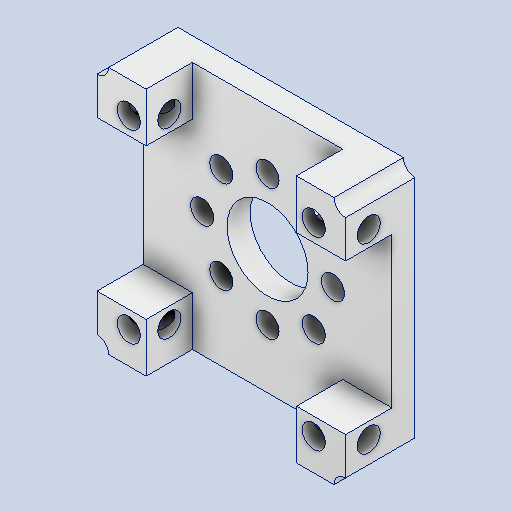
# Autodesk Inventor part: ShoulderMotorMount
Saved by Autodesk Inventor 2023 (Build 270158000, 158)
## iProperties
Created: 2021-01-26
Part Number: ShoulderMotorMount
Material: Aluminum 6061
Document SubType Name: Modeling
Designer: valer
Density: 2.7 g/cm^3
Appearance: Aluminum - Flat
Mass: 20.7246 g
Surface Area: 60.4791 cm^2
Volume: 7.6758 cm^3
Author: valer
Autodesk Inventor part; units mm, degrees
ref_plane "YZ Plane" through (0, 0, 0) normal (1, 0, 0) x (0, 1, 0)
ref_plane "XZ Plane" through (0, 0, 0) normal (0, 1, 0) x (-1, 0, 0)
ref_plane "XY Plane" through (0, 0, 0) normal (0, 0, 1) x (1, 0, 0)
sketch "Sketch1" plane through (0, 0, 0) normal (0, 0, 1) x (1, 0, 0)
  circle A0 centre (0, 0) radius 7
  line L0 (-21.5, 21.5) -> (21.5, 21.5)
  line L1 (21.5, 21.5) -> (21.5, -21.5)
  line L2 (21.5, -21.5) -> (-21.5, -21.5)
  line L3 (-21.5, -21.5) -> (-21.5, 21.5)
  line L4 (0, 0) -> (0, 21.5) construction
  line L5 (0, 0) -> (21.5, 0) construction
  dimension "d0" = 14
  dimension "d1" = 43
  constraints: 12 end point, 4 perpendicular, 2 midpoint, 2 parallel, 1 centre point, 1 coincident, 1 horizontal
  measures "d0" diameter of A0
  measures "d1" distance of L0.start L0.end
extrude "Extrusion1" add sketch "Sketch1" along normal blind 4
sketch "Sketch2" plane through (0, 0, 4) normal (0, 0, 1) x (1, 0, 0)
  line L0 (21.5, 21.5) -> (-21.5, 21.5) construction
  line L1 (-21.5, 21.5) -> (-13, 21.5)
  line L2 (-13, 21.5) -> (-13, 13)
  line L3 (-13, 13) -> (-21.5, 13)
  line L4 (-21.5, 13) -> (-21.5, 21.5)
  line L5 (0, 21.5) -> (0, -21.5) construction
  line L6 (-21.5, -21.5) -> (21.5, -21.5) construction
  line L7 (-21.5, 21.5) -> (-21.5, -21.5) construction
  line L8 (-21.5, 0) -> (21.5, 0) construction
  line L9 (21.5, -21.5) -> (21.5, 21.5) construction
  line L10 (21.5, 21.5) -> (13, 21.5)
  line L11 (13, 21.5) -> (13, 13)
  line L12 (13, 13) -> (21.5, 13)
  line L13 (21.5, 13) -> (21.5, 21.5)
  line L14 (-21.5, -21.5) -> (-13, -21.5)
  line L15 (-13, -21.5) -> (-13, -13)
  line L16 (-13, -13) -> (-21.5, -13)
  line L17 (-21.5, -13) -> (-21.5, -21.5)
  line L18 (13, -13) -> (21.5, -13)
  line L19 (13, -21.5) -> (13, -13)
  line L20 (21.5, -21.5) -> (13, -21.5)
  line L21 (21.5, -13) -> (21.5, -21.5)
  point P0 (0, 0)
  dimension "d4" = 8.5
  constraints: 36 end point, 9 symmetric about line, 4 midpoint, 2 parallel, 2 perpendicular, 1 horizontal
  measures "d4" distance of L1.end L2.end
extrude "Extrusion2" add sketch "Sketch2" along normal blind 8
sketch "Sketch3" plane through (0, 0, 4) normal (0, 0, 1) x (1, 0, 0)
  line L0 (0, 11.3137) -> (0, -11.3137) construction
  circle A0 centre (0, 11.3137) radius 2
  circle A1 centre (0, -11.3137) radius 2
  line L1 (-11.3137, 0) -> (11.3137, 0) construction
  circle A2 centre (-11.3137, 0) radius 2
  circle A3 centre (11.3137, 0) radius 2
  line L2 (-8, 8) -> (8, 8) construction
  line L3 (8, 8) -> (8, -8) construction
  line L4 (8, -8) -> (-8, -8) construction
  line L5 (-8, -8) -> (-8, 8) construction
  circle A4 centre (-8, 8) radius 2
  circle A5 centre (8, 8) radius 2
  circle A6 centre (8, -8) radius 2
  circle A7 centre (-8, -8) radius 2
  circle A8 centre (0, 0) radius 11.3137 construction
  dimension "d8" = 4
  dimension "d9" = 16
  dimension "d10" = 16
  constraints: 12 end point, 10 coincident, 9 centre point, 7 equal radius, 3 perpendicular, 3 point on circle, 2 horizontal, 2 midpoint, 2 parallel, 1 vertical
  measures "d8" diameter of A0
  measures "d9" distance of L1.start L0.start
  measures "d10" distance of L2.start L2.end
extrude "Extrusion3" cut sketch "Sketch3" against normal blind 8
sketch "Sketch4" plane through (0, 0, 12) normal (0, 0, 1) x (1, 0, 0)
  line L0 (-13, -21.5) -> (-13, -13) projected
  line L1 (-13, -13) -> (-21.5, -13) projected
  line L2 (-21.5, -13) -> (-21.5, -21.5) projected
  line L3 (-21.5, -21.5) -> (-13, -21.5) projected
  line L4 (13, -13) -> (13, -21.5) projected
  line L5 (13, -21.5) -> (21.5, -21.5) projected
  line L6 (21.5, -21.5) -> (21.5, -13) projected
  line L7 (21.5, -13) -> (13, -13) projected
  line L8 (13, 21.5) -> (13, 13) construction
  line L9 (13, 13) -> (21.5, 13) construction
  line L10 (21.5, 13) -> (21.5, 21.5) construction
  line L11 (21.5, 21.5) -> (13, 21.5) construction
  line L12 (-21.5, 13) -> (-13, 13) construction
  line L13 (-13, 13) -> (-13, 21.5) construction
  line L14 (-13, 21.5) -> (-21.5, 21.5) construction
  line L15 (-21.5, 21.5) -> (-21.5, 13) construction
  circle A0 centre (-16, -16) radius 2
  circle A1 centre (16, -16) radius 2
  line L16 (-16, -16) -> (16, -16) construction
  line L17 (0, -30.1) -> (0, 30.1) construction
  circle A2 centre (0, -11.3137) radius 2 projected
  line L18 (-21.5, 21.5) -> (-21.5, -21.5) construction
  line L19 (-21.5, 0) -> (21.5, 0) construction
  circle A3 centre (-16, 16) radius 2
  circle A4 centre (16, 16) radius 2
  circle A5 centre (-21.5, 21.5) radius 2
  circle A6 centre (21.5, 21.5) radius 2
  line L20 (-21.5, -13) -> (-21.5, -21.5) projected
  circle A7 centre (-21.5, -21.5) radius 2
  circle A8 centre (21.5, -21.5) radius 2
  point P0 (0, 0)
  point P1 (0, -16)
  dimension "d13" = 32
  dimension "d14" = 3
  dimension "d15" = 3
  constraints: 8 centre point, 6 equal radius, 4 coincident, 4 end point, 2 horizontal, 2 midpoint, 2 symmetric about line, 1 point on line, 2 other
  measures "d13" distance of L16.start L16.end
  measures "d14" distance from line of L4 L16.end
  measures "d15" distance from line of L7 L16.end
extrude "Extrusion4" cut sketch "Sketch4" against normal through all contours A7 L2 L3 | L3 L2 A7 | A8 L6 L5 | L5 L6 A8 | A0 | A1 | A3 | A4 | A5 | A6
sketch "Sketch5" plane through (-21.5, -13, 4) normal (-1, 0, 0) x (0, 0, 1)
  circle A0 centre (4, 29.25) radius 2
  circle A1 centre (4, -2.75) radius 2
  line L0 (4, 29.25) -> (4, -2.75) construction
  line L1 (8, 31) -> (8, 27) projected
  line L2 (4, 29.25) -> (8, 29.25) construction
  line L3 (8, 32.5) -> (8, 26) projected
  line L4 (4, 29.25) -> (4, 26) construction
  line L5 (0, 26) -> (8, 26) projected
  point P0 (-4, 13)
  dimension "d18" = 4
  dimension "d19" = 32
  constraints: 6 end point, 2 centre point, 2 midpoint, 2 perpendicular, 1 equal radius, 1 vertical
  measures "d18" diameter of A0
  measures "d19" distance of L0.start L0.end
extrude "Extrusion5" cut sketch "Sketch5" against normal through all contours A1
mirror "Mirror1" about plane through (0, 0, 0) normal (0, 1, 0) of "Extrusion5"
equation "\"d15\" = d14"
body "Solid1"
